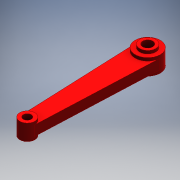
# Autodesk Inventor part: Connector_Rod
Saved by Autodesk Inventor 2016 (Build 200138000, 138)
## iProperties
Created: 2017-07-15
Part Number: Connector_Rod
Material: Steel, Carbon
Document SubType Name: Modeling
Designer: bobbyl
Density: 7.85 g/cm^3
Appearance: Red
Mass: 235.803 g
Surface Area: 103.934 cm^2
Volume: 30.0386 cm^3
Author: bobbyl
Autodesk Inventor part; units mm, degrees
ref_plane "YZ Plane" through (0, 0, 0) normal (1, 0, 0) x (0, 1, 0)
ref_plane "XZ Plane" through (0, 0, 0) normal (0, 1, 0) x (-1, 0, 0)
ref_plane "XY Plane" through (0, 0, 0) normal (0, 0, 1) x (1, 0, 0)
sketch "Sketch1" plane through (0, 0, 0) normal (0, 0, 1) x (1, 0, 0)
  line L0 (-17.5, 0) -> (17.5, 0) projected
  line L1 (0, -95.0833) -> (0, 100.9167) projected
  arc A0 (12.4891, 59.8958) -> (-12.4891, 59.8958) centre (0, 60.4167) ccw
  arc A1 (-7.4935, -59.8958) -> (7.4935, -59.8958) centre (0, -59.5833) ccw
  line L2 (-12.4891, 59.8958) -> (-7.4935, -59.8958)
  line L3 (12.4891, 59.8958) -> (7.4935, -59.8958)
  point P0 (0, 0)
  point P1 (-9.9913, 0)
  dimension "d0" = 25
  dimension "d1" = 15
  dimension "d2" = 120
  constraints: 4 end point, 4 point on circle, 4 tangent, 3 point on line, 2 centre point, 1 midpoint
  measures "d0" diameter of A0
  measures "d1" diameter of A1
  measures "d2" distance of A1.centre A0.centre
extrude "Extrusion1" add sketch "Sketch1" along normal mid plane 10
sketch "Sketch2" plane through (0, 0, 0) normal (0, 0, 1) x (1, 0, 0)
  line L0 (-7.4935, -59.8958) -> (-12.4891, 59.8958) projected
  arc A0 (12.4891, 59.8958) -> (-12.4891, 59.8958) centre (0, 60.4167) ccw projected
  line L1 (12.4891, 59.8958) -> (7.4935, -59.8958) projected
  arc A1 (-7.4935, -59.8958) -> (7.4935, -59.8958) centre (0, -59.5833) ccw projected
  circle A2 centre (0, 60.4167) radius 12.5
  circle A3 centre (0, -59.5833) radius 7.5
  point P0 (0, 0)
  constraints: 2 centre point, 2 coincident, 2 concentric
extrude "Extrusion2" add sketch "Sketch2" along normal mid plane 16 contours A3 A1 | A0 A2
sketch "Sketch3" plane through (0, 0, 0) normal (0, 0, 1) x (1, 0, 0)
  circle A0 centre (0, 60.4167) radius 8
  circle A1 centre (0, 60.4167) radius 12.5 projected
  point P0 (0, 0)
  dimension "d7" = 16
  constraints: 1 centre point, 1 concentric
  measures "d7" diameter of A0
extrude "Extrusion3" add sketch "Sketch3" along normal mid plane 22 contours A0
sketch "Sketch4" plane through (0, 0, 0) normal (0, 0, 1) x (1, 0, 0)
  arc A0 (7.4935, -59.8958) -> (-7.4935, -59.8958) centre (0, -59.5833) ccw projected
  line L0 (-7.4935, -59.8958) -> (-12.4891, 59.8958) projected
  arc A1 (-12.4891, 59.8958) -> (12.4891, 59.8958) centre (0, 60.4167) ccw projected
  line L1 (12.4891, 59.8958) -> (7.4935, -59.8958) projected
  circle A2 centre (0, 60.4167) radius 8 projected
  circle A3 centre (0, 60.4167) radius 12.5 projected
  circle A4 centre (0, -59.5833) radius 7.5 projected
  circle A5 centre (0, 60.4167) radius 5
  circle A6 centre (0, -59.5833) radius 4
  point P0 (0, 0)
  dimension "d10" = 10
  dimension "d11" = 8
  constraints: 2 centre point, 2 concentric
  measures "d10" diameter of A5
  measures "d11" diameter of A6
extrude "Extrusion4" cut sketch "Sketch4" along normal through all both and the other way through all contours A5 | A6
body "Solid1"
